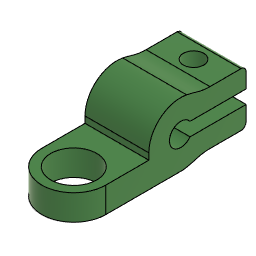
optic-fiber_1_4_20in_screw_mount v3 (Autodesk Fusion 360 design; units mm, degrees)
Autodesk Fusion 360 part; units mm, degrees
sketch "Sketch1" plane through (0, 0, 0) normal (0, 0, 1) x (1, 0, 0)
  circle A0 centre (0, 0) radius 3.429
  circle A1 centre (0, 0) radius 4.7625
  line L0 (-4.7625, 0) -> (-4.7625, 15.9606)
  line L1 (-4.7625, 15.9606) -> (4.7625, 15.9606)
  line L2 (4.7625, 15.9606) -> (4.7625, 0)
  line L3 (-4.7625, 15.9606) -> (4.7625, 15.9606)
  line L4 (4.7625, 15.9606) -> (4.7625, 6.4356)
  line L5 (4.7625, 6.4356) -> (-4.7625, 6.4356)
  line L6 (-4.7625, 6.4356) -> (-4.7625, 15.9606)
  dimension "d3" = 6.858
  dimension "d4" = 9.525
  dimension "d9" = 9.525
  constraint coincident A0.centre A1.centre
  constraint coincident A1 L0.start
  constraint tangent A1 L0
  constraint vertical L0
  constraint perpendicular L0 L1
  constraint coincident A1 L2.end
  constraint tangent A1 L2
  constraint vertical L2
  constraint horizontal L3
  constraint vertical L4
  constraint horizontal L5
  constraint vertical L6
  constraint coincident L2 L4.end
  measures "d3" diameter of A0
  measures "d4" diameter of A1
  measures "d9" distance of L0.end L5.end
extrude "Extrude1" add sketch "Sketch1" along normal blind 3.81 contours A1 | A1 L0 L2 L5
extrude "Extrude2" add sketch "Sketch1" along normal blind 9.525 contours L0 L1 L2 L3 L4 L5 L6
sketch "Sketch2" plane through (-4.7625, 0, 0) normal (-1, 0, 0) x (0, -1, 0)
  line L0 (-15.9606, 0) -> (0, 0)
  line L1 (0, 0) -> (0, 3.81)
  line L2 (0, 3.81) -> (-6.4356, 3.81)
  line L3 (-6.4356, 3.81) -> (-6.4356, 9.525)
  line L4 (-6.4356, 9.525) -> (-15.9606, 9.525)
  line L5 (-15.9606, 9.525) -> (-15.9606, 0)
  line L6 (-15.9606, 0) -> (-6.4356, 9.525) construction
  circle A0 centre (-11.1981, 4.7625) radius 1.7
  circle A1 centre (-11.1981, 4.7625) radius 4.7625
  line L7 (-6.4356, 3.81) -> (-6.4356, 9.525) construction
  line L8 (-6.4356, 4.7625) -> (-15.9606, 4.7625) construction
  line L9 (-12.5729, 5.7625) -> (-20.9378, 5.7625)
  line L10 (-20.9378, 5.7625) -> (-20.9378, 8.0005)
  line L11 (-20.1758, 8.7625) -> (-13.783, 8.7625)
  line L12 (-12.5729, 3.7625) -> (-20.9378, 3.7625)
  line L13 (-20.9378, 3.7625) -> (-20.9378, 1.5245)
  line L14 (-20.1758, 0.7625) -> (-13.783, 0.7625)
  spline S0 degree 5 poles (-12.0483, 9.4485) (-12.1187, 9.4357) (-12.2593, 9.4082) (-12.4694, 9.3611) (-12.7483, 9.2879) (-13.0955, 9.1859) (-13.4424, 9.0823) (-13.7898, 8.986) (-14.1385, 8.9039) (-14.4884, 8.8395) (-14.8393, 8.7939) (-15.1206, 8.7723) (-15.3317, 8.7643) (-15.4724, 8.7625) (-15.5428, 8.7625) knots 0 0 0 0 0 0 0.1 0.2 0.3 0.4 0.5 0.6 0.7 0.8 0.9 1 1 1 1 1 1
  spline S1 degree 5 poles (-12.0483, 0.0765) (-12.1187, 0.0893) (-12.2593, 0.1168) (-12.4694, 0.1639) (-12.7483, 0.2371) (-13.0955, 0.3391) (-13.4424, 0.4427) (-13.7898, 0.539) (-14.1385, 0.6211) (-14.4884, 0.6855) (-14.8393, 0.7311) (-15.1206, 0.7527) (-15.3317, 0.7607) (-15.4724, 0.7625) (-15.5428, 0.7625) knots 0 0 0 0 0 0 0.1 0.2 0.3 0.4 0.5 0.6 0.7 0.8 0.9 1 1 1 1 1 1
  line L15 (-11.7092, 9.51) -> (-12.3874, 9.387)
  line L16 (-15.1982, 8.7625) -> (-15.8875, 8.7625)
  line L17 (-11.7092, 0.015) -> (-12.3874, 0.138)
  line L18 (-15.1982, 0.7625) -> (-15.8875, 0.7625)
  arc A2 (-20.1758, 8.7625) -> (-20.9378, 8.0005) centre (-20.1758, 8.0005) ccw
  arc A3 (-20.9378, 1.5245) -> (-20.1758, 0.7625) centre (-20.1758, 1.5245) ccw
  point P0 (-15.9606, 0)
  point P1 (-6.4356, 9.525)
  point P2 (-20.9378, 8.7625)
  point P3 (-13.7976, 8.9876)
  point P4 (-13.7976, 0.5374)
  dimension "d14" = 3.4
  dimension "d24" = 2
  dimension "d25" = 3
  dimension "d26" = 5.395
  dimension "d27" = 0.762
  constraint coincident P0 L0.start
  constraint coincident P1 L3.end
  constraint midpoint L6 A0.centre
  constraint concentric A0 A1
  constraint tangent L3 A1
  constraint coincident L3 L8.start
  constraint coincident L5 L8.end
  constraint coincident A0.centre L8
  constraint horizontal L8
  constraint coincident A0 L9.start
  constraint horizontal L9
  constraint perpendicular L9 L10
  constraint coincident A1 L11.end
  constraint perpendicular L10 L11
  constraint symmetric L8 L9.start L12.start
  constraint symmetric L8 L9.end L12.end
  constraint symmetric L8 L11.end L14.end
  constraint coincident A1 S0.start
  constraint coincident L11 S0.end
  constraint tangent A1 S0
  constraint midpoint S0.start L15
  constraint midpoint S0.end L16
  constraint symmetric L8 S0.start S1.start
  constraint symmetric L8 P3 P4
  constraint symmetric L8 S0.end S1.end
  constraint symmetric L8 L15.start L17.start
  constraint symmetric L8 L15.end L17.end
  constraint symmetric L8 L16.start L18.start
  constraint symmetric L8 L16.end L18.end
  constraint coincident P2 L11
  constraint coincident P2 L10
  constraint tangent L11 A2
  constraint tangent L10 A2
  constraint tangent L14 A3
  constraint tangent L13 A3
  constraint equal A2 A3
  measures "d14" diameter of A0
  measures "d24" distance of L9 L12
  measures "d25" distance of L9.end P2
  measures "d26" distance of P2 S0.end
  measures "d27" radius of A2
extrude "Extrude3" cut sketch "Sketch2" against normal blind 9.525 contours L0 L5 A1 L14 S1 L18 | L3 L4 A1 | L5 A1 L12 | L4 L5 A1 L11 S0 L16 | L5 A1 L9 | A0 A1 L9 L12 | A0 picked at (-14.8762, 4.0881)
extrude "Extrude4" add sketch "Sketch2" against normal blind 9.525 contours L5 L12 L13 L14 A3 | L5 L9 L10 L11 A2
sketch "Sketch3" plane through (0, 0, 8.7625) normal (0, 0, 1) x (-1, 0, 0)
  line L0 (4.7625, -20.1758) -> (4.7625, -15.5428)
  line L1 (4.7625, -15.5428) -> (-4.7625, -15.5428)
  line L2 (-4.7625, -15.5428) -> (-4.7625, -20.1758)
  line L3 (-4.7625, -20.1758) -> (4.7625, -20.1758)
  line L4 (4.7625, -20.1758) -> (-4.7625, -15.5428) construction
  circle A0 centre (0, -17.8593) radius 1.524
  circle A1 centre (0, -17.8593) radius 1.1303
  point P0 (4.7625, -20.1758)
  point P1 (-4.7625, -15.5428)
  point P2 (0, -17.8593)
  dimension "d30" = 3.048
  dimension "d31" = 2.2606
  constraint coincident P0 L0.start
  constraint coincident P1 L1.end
  constraint midpoint L4 P2
  constraint coincident P2 A0.centre
  constraint concentric A0 A1
  measures "d30" diameter of A0
  measures "d31" diameter of A1
extrude "Extrude5" cut sketch "Sketch3" against normal blind 8.001 contours A1
extrude "Extrude6" cut sketch "Sketch3" against normal blind 3.556 contours A0
fillet "Fillet2" radius 0.635 1 edges at (-4.7625, 9.4981, 4.7625)
equation "screw_1_4_20_free_fit = 0.27 in"
equation "screw_1_4_20_cap = 0.375 in"
equation "d3 = screw_1_4_20_free_fit"
equation "d4 = screw_1_4_20_cap"
equation "optic_fiber_diam = 3 mm"
equation "optic_fiber_plastic_clearance = 0.2 mm"
equation "optic_fiber_hole_diam = optic_fiber_diam + optic_fiber_plastic_clearance * 2"
equation "screw_side_thick = 0.15 in"
equation "d9 = screw_1_4_20_cap"
equation "d10 = screw_side_thick"
equation "d12 = screw_1_4_20_cap"
equation "d14 = optic_fiber_hole_diam"
equation "clamp_thick = 3 mm"
equation "clamp_gap = 2 mm"
equation "screw_4_40_cap = 0.177 in"
equation "screw_4_40_free_fit = 0.12 in"
equation "screw_4_40_tap = 0.089 in"
equation "d24 = clamp_gap"
equation "d25 = clamp_thick"
equation "d26 = screw_4_40_cap * 1.2"
equation "d30 = screw_4_40_free_fit"
equation "d31 = screw_4_40_tap"
named bodies: "optic-fiber_1_4_20in_screw_mount_3mm"
